012 (Autodesk Fusion 360 design; units mm, degrees)
Autodesk Fusion 360 part; units mm, degrees
sketch "Esquisse1" plane through (0, 0, 0) normal (1, 0, 0) x (0, 1, 0)
  line L0 (-15, 7.5) -> (15, 7.5)
  line L1 (15, 7.5) -> (15, -7.5)
  line L2 (15, -7.5) -> (-15, -7.5)
  line L3 (-15, -7.5) -> (-15, 7.5)
  line L4 (0, 1.75) -> (0, 22.5)
  line L5 (1.75, 0) -> (22.5, 0)
  dimension "d1" = 30
  dimension "d2" = 15
  constraint horizontal L0
  constraint vertical L1
  constraint horizontal L2
  constraint vertical L3
  constraint symmetric L1 L3 L4
  constraint symmetric L0 L2 L5
  measures "d1" distance of L0.start L0.end
  measures "d2" distance of L0.start L2.end
extrude "Extrusion1" add sketch "Esquisse1" against normal blind 4
sketch "Esquisse2" plane through (0, 0, 0) normal (1, 0, 0) x (0, 1, 0)
  line L0 (-15, -7.5) -> (15, -7.5)
  line L1 (15, -7.5) -> (15, 7.5)
  line L2 (15, 7.5) -> (-15, 7.5)
  line L3 (-15, 7.5) -> (-15, -7.5)
  circle A0 centre (0, 0) radius 5.85
  dimension "d5" = 11.7
  constraint coincident A0.centre origin
  measures "d5" diameter of A0
extrude "Extrusion2" add sketch "Esquisse2" along normal blind 3 contours A0
sketch "Esquisse3" plane through (0, 0, 0) normal (1, 0, 0) x (0, 1, 0)
  circle A0 centre (0, 0) radius 5.85
  line L0 (-15, -7.5) -> (15, -7.5)
  line L1 (15, -7.5) -> (15, 7.5)
  line L2 (15, 7.5) -> (-15, 7.5)
  line L3 (-15, 7.5) -> (-15, -7.5)
  point P0 (-12, 0)
  dimension "d8" = 12
  dimension "d9" = 7.5
  measures "d8" distance of A0.centre P0
  measures "d9" distance of L2 P0
hole "Perçage1" at (0, -12, 0) direction (-1, 0, 0) diameter 3.5 depth 16 tip angle 118
mirror "Symétrie miroir1" about plane through (0, 0, 0) normal (0, 1, 0) of "Perçage1"
sketch "Esquisse4" plane through (-4, 0, 0) normal (-1, 0, 0) x (0, -1, 0)
  circle A0 centre (-12, 0) radius 1.75
  circle A1 centre (12, 0) radius 1.75
  line L0 (-15, -7.5) -> (15, -7.5)
  line L1 (15, -7.5) -> (15, 7.5)
  line L2 (15, 7.5) -> (-15, 7.5)
  line L3 (-15, 7.5) -> (-15, -7.5)
  circle A2 centre (0, 0) radius 5
  dimension "d15" = 10
  constraint coincident A2.centre origin
  measures "d15" diameter of A2
extrude "Extrusion3" add sketch "Esquisse4" along normal blind 50 contours A2
fillet "Congé1" radius 2 1 edges at (-54, 4.6616, -1.8081)
sketch "Esquisse5" plane through (-54, 0, 0) normal (-1, 0, 0) x (0, -1, 0)
  circle A0 centre (0, 0) radius 3
  circle A1 centre (0, 0) radius 1.1
  dimension "d20" = 2.2
  constraint coincident A0.centre A1.centre
  measures "d20" diameter of A1
extrude "Extrusion4" cut sketch "Esquisse5" against normal blind 14 contours A1
sketch "Esquisse6" plane through (0, 0, 0) normal (0, 1, 0) x (1, 0, 0)
  circle A0 centre (-5.3907, 0) radius 1
  dimension "d23" = 2
  measures "d23" diameter of A0
extrude "Extrusion5" cut sketch "Esquisse6" along normal mid plane 18
sketch "Esquisse7" plane through (0, 0, 0) normal (0, 0, 1) x (1, 0, 0)
  circle A0 centre (-5.5, 0) radius 1.25
  line L0 (1.75, 0) -> (22.5, 0)
  dimension "d26" = 2.5
  dimension "d27" = 5.5
  constraint coincident A0.centre L0
  measures "d26" diameter of A0
  measures "d27" distance of origin A0.centre
extrude "Extrusion6" cut sketch "Esquisse7" along normal blind 5.5
fillet "Congé2" [no effect]
fillet "Congé3" [no effect]
